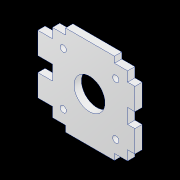
# Autodesk Inventor part: DriveSideFrame_02
Saved by Autodesk Inventor 2021 (Build 250183000, 183)
## iProperties
Created: 2021-03-08
Part Number: DriveSideFrame_02
Material: Aluminum 6061
Document SubType Name: Modeling
Designer: M3rob
Density: 2.7 g/cm^3
Appearance: Aluminum - Flat
Mass: 285.486 g
Surface Area: 295.726 cm^2
Volume: 105.736 cm^3
Author: M3rob
Autodesk Inventor part; units mm, degrees
ref_plane "YZ Plane" through (0, 0, 0) normal (1, 0, 0) x (0, 1, 0)
ref_plane "XZ Plane" through (0, 0, 0) normal (0, 1, 0) x (-1, 0, 0)
ref_plane "XY Plane" through (0, 0, 0) normal (0, 0, 1) x (1, 0, 0)
sketch "Sketch1" plane through (0, 0, 0) normal (0, 0, 1) x (1, 0, 0)
  line L0 (-48.895, 50.8) -> (-48.895, 38.1)
  line L1 (-48.895, -50.8) -> (-31.75, -50.8)
  line L2 (48.895, -50.8) -> (48.895, -38.1)
  line L3 (48.895, 50.8) -> (31.75, 50.8)
  line L4 (-48.895, 0) -> (48.895, 0) construction
  line L5 (48.895, 38.1) -> (58.42, 38.1)
  line L6 (58.42, 38.1) -> (58.42, 9.525)
  line L7 (58.42, 9.525) -> (48.895, 9.525)
  line L8 (48.895, -9.525) -> (58.42, -9.525)
  line L9 (58.42, -9.525) -> (58.42, -38.1)
  line L10 (58.42, -38.1) -> (48.895, -38.1)
  line L11 (48.895, 38.1) -> (48.895, 50.8)
  line L12 (48.895, 9.525) -> (48.895, 38.1) construction
  line L13 (48.895, -9.525) -> (48.895, 9.525)
  line L14 (48.895, -38.1) -> (48.895, -9.525) construction
  line L15 (-48.895, 6.7437) -> (-39.37, 6.7437) construction
  line L16 (-39.37, 6.7437) -> (-39.37, 9.525) construction
  line L17 (-39.37, 9.525) -> (-31.4325, 9.525) construction
  line L18 (-31.4325, 9.525) -> (-31.4325, 6.7437) construction
  line L19 (-31.4325, 6.7437) -> (-28.2575, 6.7437) construction
  line L20 (-28.2575, 6.7437) -> (-28.2575, -6.7437) construction
  line L21 (-28.2575, -6.7437) -> (-31.4325, -6.7437) construction
  line L22 (-31.4325, -6.7437) -> (-31.4325, -9.525) construction
  line L23 (-31.4325, -9.525) -> (-39.37, -9.525) construction
  line L24 (-39.37, -9.525) -> (-39.37, -6.7437) construction
  line L25 (-39.37, -6.7437) -> (-48.895, -6.7437) construction
  line L26 (-48.895, 6.7437) -> (-48.895, -6.7437)
  line L27 (-48.895, -6.7437) -> (-48.895, -9.525)
  line L28 (-31.75, 50.8) -> (-31.75, 58.7375)
  line L29 (-31.75, 58.7375) -> (31.75, 58.7375)
  line L30 (31.75, 58.7375) -> (31.75, 50.8)
  line L31 (-31.75, -50.8) -> (-31.75, -58.7375)
  line L32 (-31.75, -58.7375) -> (31.75, -58.7375)
  line L33 (31.75, -58.7375) -> (31.75, -50.8)
  line L34 (-31.75, 50.8) -> (-48.895, 50.8)
  line L35 (31.75, 50.8) -> (-31.75, 50.8) construction
  line L36 (31.75, -50.8) -> (48.895, -50.8)
  line L37 (-31.75, -50.8) -> (31.75, -50.8) construction
  line L38 (-48.895, 38.1) -> (-67.945, 38.1)
  line L39 (-67.945, 38.1) -> (-67.945, 9.525)
  line L40 (-67.945, 9.525) -> (-48.895, 9.525)
  line L41 (-48.895, -9.525) -> (-67.945, -9.525)
  line L42 (-67.945, -9.525) -> (-67.945, -38.1)
  line L43 (-67.945, -38.1) -> (-48.895, -38.1)
  line L44 (-48.895, 38.1) -> (-48.895, 9.525) construction
  line L45 (-48.895, 9.525) -> (-48.895, 6.7437)
  line L46 (-48.895, -9.525) -> (-48.895, -38.1) construction
  line L47 (-48.895, -38.1) -> (-48.895, -50.8)
  circle A0 centre (-0.635, 0) radius 7.9375
  circle A1 centre (-0.635, 0) radius 20.066
  point P0 (0, 0)
  point P1 (0, 0)
  point P2 (0, 58.7375)
  point P3 (0, -58.7375)
  point P4 (58.42, 23.8125)
  point P5 (-96.52, 6.35)
  point P6 (-96.52, -6.35)
  dimension "d0" = 101.6
  dimension "d1" = 97.79
  dimension "d2" = 19.05
  dimension "d3" = 12.7
  dimension "d4" = 9.525
  dimension "d5" = 13.4874
  dimension "d6" = 9.525
  dimension "d7" = 7.9375
  dimension "d8" = 3.175
  dimension "d9" = 19.05
  dimension "d10" = 63.5
  dimension "d11" = 7.9375
  dimension "d12" = 19.05
  dimension "d13" = 48.26
  dimension "d14" = 15.875
  dimension "d17" = 40.132
  constraints: 96 end point, 66 perpendicular, 39 parallel, 11 point on line, 9 vertical, 6 midpoint, 3 equal length, 3 horizontal, 3 symmetric about line, 2 centre point, 2 coincident, 2 horizontal alignment, 2 vertical alignment, 7 other
  measures "d0" distance of L0.start L1.start
  measures "d1" distance of L3.start L0.start
  measures "d2" diameter of L7 L4
  measures "d3" distance of L3.start L5.start
  measures "d4" distance of L5.start L5.end
  measures "d5" distance between parallel lines of L25 L15
  measures "d6" distance of L15.start L15.end
  measures "d7" distance of L16.end L17.end
  measures "d8" distance of L18.end L19.end
  measures "d9" distance between parallel lines of L23 L17
  measures "d10" distance of L28.end L29.end
  measures "d11" distance of L32.end L33.end
  measures "d12" distance of L0.end L38.end
  measures "d13" horizontal distance of L27.end A0.centre
  measures "d14" diameter of A0
  measures "d17" diameter of A1
extrude "Extrusion2" add sketch "Sketch1" along normal blind 9.525 contours L34 L28 L29 L30 L3 L11 L5 L6 L7 L13 L8 L9 L10 L2 L36 L33 L32 L31 L1 L47 L43 L42 L41 L27 L26 L45 L40 L39 L38 L0
sketch "Sketch2" plane through (0, 0, 9.525) normal (0, 0, 1) x (1, 0, 0)
  circle A0 centre (-0.635, 0) radius 27.8049
  circle A1 centre (-0.635, 0) radius 20.066 projected
  line L0 (-34.798, -34.163) -> (33.528, -34.163) construction
  line L1 (33.528, -34.163) -> (-34.798, -34.163) construction
  line L2 (-34.798, -34.163) -> (-34.798, 34.163) construction
  line L3 (-34.798, 34.163) -> (33.528, 34.163) construction
  line L4 (33.528, 34.163) -> (33.528, -34.163) construction
  line L5 (33.528, -34.163) -> (-34.798, 34.163) construction
  line L6 (-34.798, -34.163) -> (33.528, 34.163) construction
  point P0 (-0.635, 27.9401)
  point P1 (-41.9049, 0)
  dimension "d34" = 68.326
  dimension "d35" = 68.326
  constraints: 14 end point, 2 horizontal, 2 midpoint, 2 parallel, 1 centre point, 1 coincident, 1 concentric, 1 horizontal alignment, 1 perpendicular, 1 vertical alignment
  measures "d34" distance of L2.end L3.end
  measures "d35" distance of L0.start L2.end
hole "Hole1" at (-34.798, 34.163, 9.525) at (33.528, 34.163, 9.525) at (-34.798, -34.163, 9.525) at (33.528, -34.163, 9.525) direction (0, 0, -1) diameter 8.1915 end through all
sketch "Sketch3" plane through (0, 0, 9.525) normal (0, 0, 1) x (1, 0, 0)
  line L0 (48.895, 50.8) -> (31.75, 50.8) projected
  line L1 (48.895, 38.1) -> (48.895, 50.8) projected
  line L2 (31.75, -50.8) -> (48.895, -50.8) projected
  line L3 (48.895, -50.8) -> (48.895, -38.1) projected
  circle A0 centre (33.528, 34.163) radius 4.0957 projected
  circle A1 centre (33.528, -34.163) radius 4.0957 projected
  line L4 (48.895, 50.8) -> (36.195, 50.8)
  line L5 (36.195, 50.8) -> (36.195, 38.1) construction
  line L6 (36.195, 38.1) -> (48.895, 38.1) construction
  line L7 (48.895, 38.1) -> (48.895, 50.8)
  line L8 (48.895, -50.8) -> (36.195, -50.8)
  line L9 (36.195, -50.8) -> (36.195, -38.1) construction
  line L10 (36.195, -38.1) -> (48.895, -38.1) construction
  line L11 (48.895, -38.1) -> (48.895, -50.8)
  line L12 (37.6238, 34.163) -> (50.3238, 34.163) construction
  line L13 (-31.75, -58.7375) -> (31.75, -58.7375) projected
  line L14 (36.195, -38.1) -> (36.195, 38.1)
  line L15 (36.195, 38.1) -> (32.131, 0) construction
  line L16 (36.195, -38.1) -> (32.131, 0) construction
  circle A2 centre (-0.635, 0) radius 20.066 projected
  line L17 (19.431, 0) -> (32.131, 0) construction
  line L18 (36.195, 0) -> (36.195, 6.35)
  line L19 (36.195, 0) -> (36.195, -6.35)
  line L20 (36.195, 6.35) -> (114.7233, 6.35) construction
  line L21 (36.195, -6.35) -> (32.8083, -6.35)
  line L22 (31.75, 50.8) -> (36.195, 50.8)
  line L23 (36.195, 50.8) -> (36.195, 38.1)
  line L24 (36.195, 38.1) -> (31.75, 38.1) construction
  line L25 (31.75, 38.1) -> (31.75, 50.8) construction
  line L26 (17.1027, 6.35) -> (17.1027, -6.35)
  line L27 (17.1027, -6.35) -> (32.8083, -6.35)
  line L28 (36.195, 6.35) -> (17.1027, 6.35)
  line L29 (26.6488, 6.35) -> (26.6488, 38.1) construction
  line L30 (26.6488, 6.35) -> (26.6488, -50.8) construction
  line L31 (31.75, -50.8) -> (48.895, -50.8) construction
  line L32 (17.1027, 6.35) -> (26.6488, 38.1)
  line L33 (36.195, 6.35) -> (26.6488, 38.1)
  line L34 (26.6488, -50.8) -> (26.6488, -38.1) construction
  line L35 (17.1027, -6.35) -> (26.6488, -38.1)
  line L36 (36.195, -6.35) -> (26.6488, -38.1)
  circle A3 centre (33.528, 34.163) radius 16.7958 construction
  line L37 (26.6488, 6.35) -> (32.9988, 6.35)
  line L38 (26.6488, 6.35) -> (20.2988, 6.35)
  line L39 (32.9988, 6.35) -> (32.9988, 16.9803)
  line L40 (20.2988, 6.35) -> (20.2988, 16.9803)
  line L41 (32.9988, 6.35) -> (32.9988, -6.35) construction
  line L42 (20.2988, 6.35) -> (20.2988, -6.35) construction
  line L43 (32.9988, -6.35) -> (32.9988, -16.9803)
  line L44 (20.2988, -6.35) -> (20.2988, -16.9803)
  point P0 (0, 0)
  dimension "d36" = 12.7
  dimension "d37" = 12.7
  dimension "d38" = 12.7
  dimension "d39" = 12.7
  dimension "d40" = 12.7
  dimension "d42" = 12.7
  dimension "d46" = 6.35
  dimension "d47" = 6.35
  dimension "d49" = 12.7
  dimension "d50" = 6.35
  dimension "d51" = 6.35
  constraints: 78 end point, 15 point on line, 9 perpendicular, 8 parallel, 7 horizontal, 3 horizontal alignment, 2 midpoint, 2 vertical, 1 coincident, 4 other
  measures "d36" distance of L6.end L5.end
  measures "d37" distance of L5.end L4.end
  measures "d38" distance of L9.end L10.end
  measures "d39" distance of L8.end L9.end
  measures "d40" distance of L12.start L12.end
  measures "d42" distance of L17.start L15.end
  measures "d46" distance of L18.start L18.end
  measures "d47" distance of L18.start L19.end
  measures "d49" distance of L30.end L34.end
  measures "d50" distance of L29.start L37.end
  measures "d51" distance of L29.start L38.end
extrude "Extrusion3" [suppressed]
fillet "Fillet1" [suppressed]
sketch "Sketch4" plane through (0, 0, 9.525) normal (0, 0, 1) x (1, 0, 0)
  circle A0 centre (-34.798, -34.163) radius 4.0957 projected
  circle A1 centre (-34.798, 34.163) radius 4.0957 projected
  circle A2 centre (33.528, 34.163) radius 4.0957 projected
  circle A3 centre (33.528, -34.163) radius 4.0957 projected
  line L0 (-48.895, 50.8) -> (-48.895, 38.1) projected
  line L1 (-48.895, 38.1) -> (-67.945, 38.1) projected
  line L2 (-67.945, 38.1) -> (-67.945, 9.525) projected
  line L3 (-67.945, 9.525) -> (-48.895, 9.525) projected
  line L4 (-48.895, 9.525) -> (-48.895, -9.525) projected
  line L5 (-48.895, -9.525) -> (-67.945, -9.525) projected
  line L6 (-67.945, -9.525) -> (-67.945, -38.1) projected
  line L7 (-67.945, -38.1) -> (-48.895, -38.1) projected
  line L8 (-48.895, -38.1) -> (-48.895, -50.8) projected
  line L9 (-48.895, -50.8) -> (-31.75, -50.8) projected
  line L10 (-31.75, -50.8) -> (-31.75, -58.7375) projected
  line L11 (-31.75, -58.7375) -> (31.75, -58.7375) projected
  line L12 (31.75, -58.7375) -> (31.75, -50.8) projected
  line L13 (31.75, -50.8) -> (48.895, -50.8) projected
  line L14 (48.895, -50.8) -> (48.895, -38.1) projected
  line L15 (48.895, -38.1) -> (58.42, -38.1) projected
  line L16 (58.42, -38.1) -> (58.42, -9.525) projected
  line L17 (58.42, -9.525) -> (48.895, -9.525) projected
  line L18 (48.895, -9.525) -> (48.895, 9.525) projected
  line L19 (48.895, 9.525) -> (58.42, 9.525) projected
  line L20 (58.42, 9.525) -> (58.42, 38.1) projected
  line L21 (58.42, 38.1) -> (48.895, 38.1) projected
  line L22 (48.895, 38.1) -> (48.895, 50.8) projected
  line L23 (48.895, 50.8) -> (31.75, 50.8) projected
  line L24 (31.75, 50.8) -> (31.75, 58.7375) projected
  line L25 (31.75, 58.7375) -> (-31.75, 58.7375) projected
  line L26 (-31.75, 58.7375) -> (-31.75, 50.8) projected
  line L27 (-31.75, 50.8) -> (-48.895, 50.8) projected
  circle A4 centre (-0.635, 0) radius 20.066 projected
  line L28 (19.05, 38.1) -> (36.195, 38.1)
  line L29 (36.195, 38.1) -> (36.195, 25.4)
  line L30 (36.195, 25.4) -> (45.72, 25.4)
  line L31 (45.72, 25.4) -> (45.72, 22.225)
  line L32 (45.72, 22.225) -> (36.195, 22.225)
  line L33 (36.195, 22.225) -> (36.195, -22.225)
  line L34 (36.195, -22.225) -> (45.72, -22.225)
  line L35 (45.72, -22.225) -> (45.72, -25.4)
  line L36 (45.72, -25.4) -> (36.195, -25.4)
  line L37 (36.195, -25.4) -> (36.195, -38.1)
  line L38 (36.195, -38.1) -> (19.05, -38.1)
  line L39 (19.05, -38.1) -> (19.05, -46.0375)
  line L40 (19.05, -46.0375) -> (-19.05, -46.0375)
  line L41 (-19.05, -46.0375) -> (-19.05, -38.1)
  line L42 (-19.05, -38.1) -> (-36.195, -38.1)
  line L43 (-36.195, -38.1) -> (-36.195, -25.4)
  line L44 (-36.195, -25.4) -> (-55.245, -25.4)
  line L45 (-55.245, -25.4) -> (-55.245, -22.225)
  line L46 (-55.245, -22.225) -> (-36.195, -22.225)
  line L47 (-36.195, -22.225) -> (-36.195, 22.225)
  line L48 (-36.195, 22.225) -> (-55.245, 22.225)
  line L49 (-55.245, 22.225) -> (-55.245, 25.4)
  line L50 (-55.245, 25.4) -> (-36.195, 25.4)
  line L51 (-36.195, 25.4) -> (-36.195, 38.1)
  line L52 (-36.195, 38.1) -> (-19.05, 38.1)
  line L53 (-19.05, 38.1) -> (-19.05, 46.0375)
  line L54 (-19.05, 46.0375) -> (19.05, 46.0375)
  line L55 (19.05, 46.0375) -> (19.05, 38.1)
  circle A5 centre (33.528, 34.163) radius 16.7958
  circle A6 centre (-34.798, 34.163) radius 16.7958
  circle A7 centre (33.528, -34.163) radius 16.7958
  circle A8 centre (-34.798, -34.163) radius 16.7958
  circle A9 centre (-0.635, 0) radius 32.766
  point P0 (0, 0)
  dimension "t" = 12.7
  dimension "d53" = 12.7
  dimension "d54" = 12.7
  dimension "d55" = 12.7
  dimension "d56" = 12.7
  dimension "d57" = 12.7
  constraints: 56 end point, 5 centre point, 27 other
  measures "t" distance between parallel lines of L23 L28
  measures "d53" radial gap between concentric circles of A2 A5
  measures "d54" radial gap between concentric circles of A1 A6
  measures "d55" radial gap between concentric circles of A3 A7
  measures "d56" radial gap between concentric circles of A0 A8
  measures "d57" radial gap between concentric circles of A4 A9
equation "\"d53\" = t"
equation "\"d54\" = t"
equation "\"d55\" = t"
equation "\"d56\" = t"
equation "\"d57\" = t"
body "Solid2"
